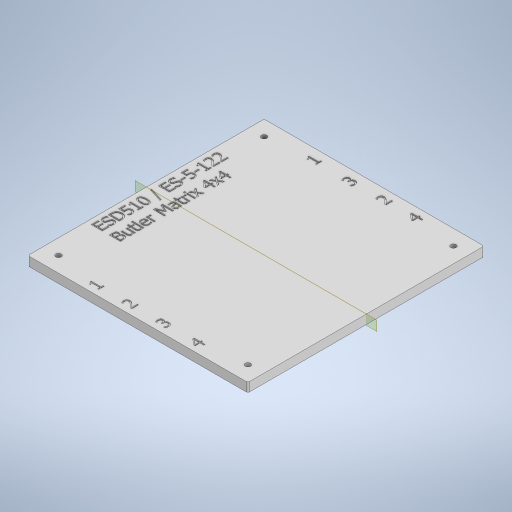
# Autodesk Inventor part: Cover_acryl
Saved by Autodesk Inventor 2023.5 (Build 275446000, 446)
## iProperties
Created: 2025-10-09
Part Number: Cover_acryl
Material: Generic
Document SubType Name: Modeling
Designer: Mikke
Density: 1 g/cm^3
Appearance: Default
Author: Mikke
Autodesk Inventor part; units mm, degrees
(part 1 of 2)
ref_plane "YZ Plane" through (0, 0, 0) normal (1, 0, 0) x (0, 1, 0)
ref_plane "XZ Plane" through (0, 0, 0) normal (0, 1, 0) x (-1, 0, 0)
ref_plane "XY Plane" through (0, 0, 0) normal (0, 0, 1) x (1, 0, 0)
sketch "Sketch1" plane through (0, 0, 0) normal (0, 1, 0) x (-1, 0, 0)
  line L0 (-61, 65.5) -> (61, 65.5)
  line L1 (61, 65.5) -> (61, -65.5)
  line L2 (61, -65.5) -> (-61, -65.5)
  line L3 (-61, -65.5) -> (-61, 65.5)
  line L4 (-61, 65.5) -> (61, -65.5) construction
  line L5 (61, 65.5) -> (-61, -65.5) construction
  point P0 (0, 0)
  dimension "d0" = 122
  dimension "d1" = 131
  constraints: 12 end point, 2 midpoint, 2 parallel, 1 horizontal, 1 perpendicular
  measures "d0" distance of L1.end L2.end
  measures "d1" distance of L0.end L1.end
extrude "Extrusion1" add sketch "Sketch1" along normal blind 5
sketch "Sketch2" plane through (0, 5, 0) normal (0, 1, 0) x (1, 0, 0)
  line L0 (-61, 65.5) -> (-61, -65.5) projected
  line L1 (-61, -65.5) -> (-52.5, -65.5)
  line L2 (-52.5, -65.5) -> (-52.5, -57)
  line L3 (-52.5, -57) -> (-61, -57)
  line L4 (-61, -57) -> (-61, -65.5)
  circle A0 centre (-52.5, -57) radius 1.5
  line L5 (-61, 65.5) -> (-61, -65.5) projected
  line L6 (-61, 65.5) -> (-52.5, 65.5)
  line L7 (-52.5, 65.5) -> (-52.5, 57)
  line L8 (-52.5, 57) -> (-61, 57)
  line L9 (-61, 57) -> (-61, 65.5)
  line L10 (61, 65.5) -> (-61, 65.5) projected
  line L11 (61, 65.5) -> (52.5, 65.5)
  line L12 (52.5, 65.5) -> (52.5, 57)
  line L13 (52.5, 57) -> (61, 57)
  line L14 (61, 57) -> (61, 65.5)
  line L15 (-61, -65.5) -> (61, -65.5) projected
  line L16 (61, -65.5) -> (52.5, -65.5)
  line L17 (52.5, -65.5) -> (52.5, -57)
  line L18 (52.5, -57) -> (61, -57)
  line L19 (61, -57) -> (61, -65.5)
  circle A1 centre (52.5, -57) radius 1.5
  circle A2 centre (52.5, 57) radius 1.5
  circle A3 centre (-52.5, 57) radius 1.5
  point P0 (0, 0)
  dimension "d4" = 8.5
  dimension "d5" = 8.5
  dimension "d6" = 3
  dimension "d7" = 8.5
  dimension "d8" = 8.5
  dimension "d9" = 8.5
  dimension "d10" = 8.5
  dimension "d11" = 8.5
  dimension "d12" = 8.5
  dimension "d13" = 3
  dimension "d14" = 3
  dimension "d15" = 3
  constraints: 32 end point, 8 parallel, 4 centre point, 4 coincident, 4 horizontal, 4 perpendicular
  measures "d4" distance of L3.end L2.end
  measures "d5" distance of L2.end L1.end
  measures "d6" diameter of A0
  measures "d7" distance of L7.end L8.end
  measures "d8" distance of L6.end L7.end
  measures "d9" distance of L13.end L12.end
  measures "d10" distance of L12.end L11.end
  measures "d11" distance of L17.end L18.end
  measures "d12" distance of L16.end L17.end
  measures "d13" diameter of A1
  measures "d14" diameter of A2
  measures "d15" diameter of A3
extrude "Extrusion2" cut sketch "Sketch2" against normal blind 5 contours A3 L7 L8 | L8 L7 A3 | A0 L2 L3 | L3 L2 A0 | A2 L13 L12 | L12 L13 A2 | A1 L18 L17 | L17 L18 A1
fillet "Fillet1" radius 1 4 edges at (61, 2.5, 65.5) (61, 2.5, -65.5) (-61, 2.5, -65.5) (-61, 2.5, 65.5)
sketch "Sketch4" plane through (0, 5, 0) normal (0, 1, 0) x (1, 0, 0)
  line L0 (-60, -65.5) -> (60, -65.5) projected
  line L1 (60, 65.5) -> (-60, 65.5) projected
  line L2 (0, -65.5) -> (-9.425, -65.5)
  line L3 (0, -65.5) -> (9.425, -65.5)
  line L4 (-9.425, -65.5) -> (-28.275, -65.5)
  line L5 (9.425, -65.5) -> (28.275, -65.5)
  line L6 (24.7297, -62.6951) -> (24.7297, -58.1177) construction
  line L7 (24.7297, -58.1177) -> (30.8297, -58.1177) construction
  line L8 (30.8297, -58.1177) -> (30.8297, -62.6951) construction
  line L9 (30.8297, -62.6951) -> (24.7297, -62.6951) construction
  line L10 (-31.1768, -63.0534) -> (-31.1768, -58.4759) construction
  line L11 (-31.1768, -58.4759) -> (-25.057, -58.4759) construction
  line L12 (-25.057, -58.4759) -> (-25.057, -63.0534) construction
  line L13 (-25.057, -63.0534) -> (-31.1768, -63.0534) construction
  line L14 (-12.8022, -62.7702) -> (-12.8022, -58.1927) construction
  line L15 (-12.8022, -58.1927) -> (-6.5737, -58.1927) construction
  line L16 (-6.5737, -58.1927) -> (-6.5737, -62.7702) construction
  line L17 (-6.5737, -62.7702) -> (-12.8022, -62.7702) construction
  line L18 (5.8471, -62.6329) -> (5.8471, -58.0555) construction
  line L19 (5.8471, -58.0555) -> (12.2041, -58.0555) construction
  line L20 (12.2041, -58.0555) -> (12.2041, -62.6329) construction
  line L21 (12.2041, -62.6329) -> (5.8471, -62.6329) construction
  line L22 (-28.275, -65.5) -> (-28.275, 65.5)
  line L23 (25.0797, 57.6837) -> (25.0797, 62.2611) construction
  line L24 (25.0797, 62.2611) -> (31.1797, 62.2611) construction
  line L25 (31.1797, 62.2611) -> (31.1797, 57.6837) construction
  line L26 (31.1797, 57.6837) -> (25.0797, 57.6837) construction
  line L27 (-30.8268, 57.3254) -> (-30.8268, 61.9029) construction
  line L28 (-30.8268, 61.9029) -> (-24.707, 61.9029) construction
  line L29 (-24.707, 61.9029) -> (-24.707, 57.3254) construction
  line L30 (-24.707, 57.3254) -> (-30.8268, 57.3254) construction
  line L31 (7.8308, 57.6086) -> (7.8308, 62.1861) construction
  line L32 (7.8308, 62.1861) -> (14.0593, 62.1861) construction
  line L33 (14.0593, 62.1861) -> (14.0593, 57.6086) construction
  line L34 (14.0593, 57.6086) -> (7.8308, 57.6086) construction
  line L35 (-10.5783, 57.1359) -> (-10.5783, 61.7133) construction
  line L36 (-10.5783, 61.7133) -> (-4.2212, 61.7133) construction
  line L37 (-4.2212, 61.7133) -> (-4.2212, 57.1359) construction
  line L38 (-4.2212, 57.1359) -> (-10.5783, 57.1359) construction
  line L39 (-25.057, -59.1531) -> (-25.057, -62.129)
  line L40 (-25.057, -62.129) -> (-25.6799, -62.129)
  line L41 (-25.6799, -62.129) -> (-25.6799, -61.0217)
  line L42 (-25.6799, -61.0217) -> (-29.768, -61.0217)
  line L43 (-29.768, -61.0217) -> (-29.768, -62.129)
  line L44 (-29.768, -62.129) -> (-30.3266, -62.129)
  spline S0 degree 2 poles (-30.3266, -62.129) (-30.3266, -61.5012) (-30.6825, -60.908) (-31.1768, -60.8684) knots 0 0 0 1 2 2 2
  line L45 (-31.1768, -60.8684) -> (-31.1768, -60.2357)
  line L46 (-31.1768, -60.2357) -> (-25.6799, -60.2357)
  line L47 (-25.6799, -60.2357) -> (-25.6799, -59.1531)
  line L48 (-25.6799, -59.1531) -> (-25.057, -59.1531)
  line L49 (-6.5737, -58.5635) -> (-6.5737, -62.3253)
  line L50 (-6.5737, -62.3253) -> (-7.4388, -62.3253)
  spline S1 degree 2 poles (-7.4388, -62.3253) (-7.8194, -61.9199) (-8.5263, -61.1982) (-8.9069, -60.8522) knots 0 0 0 1 2 2 2
  spline S2 degree 2 poles (-8.9069, -60.8522) (-9.6731, -60.1552) (-10.5926, -59.646) (-11.0819, -59.646) knots 0 0 0 1 2 2 2
  spline S3 degree 2 poles (-11.0819, -59.646) (-11.339, -59.646) (-11.7246, -59.8042) (-11.8482, -59.9476) knots 0 0 0 1 2 2 2
  spline S4 degree 2 poles (-11.8482, -59.9476) (-11.9717, -60.0909) (-12.0953, -60.4666) (-12.0953, -60.694) knots 0 0 0 1 2 2 2
  spline S5 degree 2 poles (-12.0953, -60.694) (-12.0953, -60.9115) (-11.9866, -61.3564) (-11.9025, -61.5591) knots 0 0 0 1 2 2 2
  spline S6 degree 2 poles (-11.9025, -61.5591) (-11.8333, -61.7321) (-11.6356, -62.0534) (-11.5664, -62.1523) knots 0 0 0 1 2 2 2
  line L51 (-11.5664, -62.1523) -> (-11.5664, -62.1968)
  line L52 (-11.5664, -62.1968) -> (-12.4364, -62.1968)
  spline S7 degree 2 poles (-12.4364, -62.1968) (-12.56, -61.9447) (-12.8022, -61.04) (-12.8022, -60.6347) knots 0 0 0 1 2 2 2
  spline S8 degree 2 poles (-12.8022, -60.6347) (-12.8022, -59.7795) (-11.8976, -58.8156) (-11.1264, -58.8156) knots 0 0 0 1 2 2 2
  spline S9 degree 2 poles (-11.1264, -58.8156) (-10.7656, -58.8156) (-10.1625, -58.9836) (-9.9054, -59.1319) knots 0 0 0 1 2 2 2
  spline S10 degree 2 poles (-9.9054, -59.1319) (-9.6385, -59.2802) (-9.1145, -59.7103) (-8.8624, -59.9476) knots 0 0 0 1 2 2 2
  spline S11 degree 2 poles (-8.8624, -59.9476) (-8.4422, -60.3331) (-7.5426, -61.2773) (-7.2806, -61.5591) knots 0 0 0 1 2 2 2
  line L53 (-7.2806, -61.5591) -> (-7.2806, -58.5635)
  line L54 (-7.2806, -58.5635) -> (-6.5737, -58.5635)
  spline S12 degree 2 poles (6.554, -60.5419) (6.554, -60.7644) (6.6627, -61.2043) (6.7467, -61.4169) knots 0 0 0 1 2 2 2
  spline S13 degree 2 poles (6.7467, -61.4169) (6.8308, -61.6146) (7.0087, -61.9063) (7.0878, -62.02) knots 0 0 0 1 2 2 2
  line L55 (7.0878, -62.02) -> (7.0878, -62.0694)
  line L56 (7.0878, -62.0694) -> (6.2228, -62.0694)
  spline S14 degree 2 poles (6.2228, -62.0694) (6.0794, -61.8025) (5.8471, -60.888) (5.8471, -60.4777) knots 0 0 0 1 2 2 2
  spline S15 degree 2 poles (5.8471, -60.4777) (5.8471, -60.0624) (6.0151, -59.4445) (6.1931, -59.1924) knots 0 0 0 1 2 2 2
  spline S16 degree 2 poles (6.1931, -59.1924) (6.3859, -58.9255) (6.9445, -58.6487) (7.3202, -58.6487) knots 0 0 0 1 2 2 2
  spline S17 degree 2 poles (7.3202, -58.6487) (7.8244, -58.6487) (8.5856, -59.3111) (8.6845, -59.7757) knots 0 0 0 1 2 2 2
  line L57 (8.6845, -59.7757) -> (8.7438, -59.7757)
  spline S18 degree 2 poles (8.7438, -59.7757) (8.7834, -59.5829) (8.9613, -59.143) (9.1393, -58.9551) knots 0 0 0 1 2 2 2
  spline S19 degree 2 poles (9.1393, -58.9551) (9.3123, -58.7673) (9.866, -58.53) (10.2664, -58.53) knots 0 0 0 1 2 2 2
  spline S20 degree 2 poles (10.2664, -58.53) (10.6767, -58.53) (11.3737, -58.8118) (11.6406, -59.0688) knots 0 0 0 1 2 2 2
  spline S21 degree 2 poles (11.6406, -59.0688) (11.9174, -59.3358) (12.2041, -60.0921) (12.2041, -60.5716) knots 0 0 0 1 2 2 2
  spline S22 degree 2 poles (12.2041, -60.5716) (12.2041, -61.0313) (11.9817, -61.931) (11.8284, -62.2375) knots 0 0 0 1 2 2 2
  line L58 (11.8284, -62.2375) -> (10.9634, -62.2375)
  line L59 (10.9634, -62.2375) -> (10.9634, -62.1782)
  spline S23 degree 2 poles (10.9634, -62.1782) (11.1512, -61.9211) (11.4972, -61.0511) (11.4972, -60.621) knots 0 0 0 1 2 2 2
  spline S24 degree 2 poles (11.4972, -60.621) (11.4972, -60.3689) (11.339, -59.8647) (11.1561, -59.6966) knots 0 0 0 1 2 2 2
  spline S25 degree 2 poles (11.1561, -59.6966) (10.9732, -59.5335) (10.5382, -59.3605) (10.207, -59.3605) knots 0 0 0 1 2 2 2
  spline S26 degree 2 poles (10.207, -59.3605) (9.8758, -59.3605) (9.4458, -59.5533) (9.3222, -59.7263) knots 0 0 0 1 2 2 2
  spline S27 degree 2 poles (9.3222, -59.7263) (9.1986, -59.8993) (9.1047, -60.3689) (9.1047, -60.6457) knots 0 0 0 1 2 2 2
  line L60 (9.1047, -60.6457) -> (9.1047, -60.9918)
  line L61 (9.1047, -60.9918) -> (8.4275, -60.9918)
  line L62 (8.4275, -60.9918) -> (8.4275, -60.7199)
  spline S28 degree 2 poles (8.4275, -60.7199) (8.4275, -60.1712) (7.9035, -59.4791) (7.4042, -59.4791) knots 0 0 0 1 2 2 2
  spline S29 degree 2 poles (7.4042, -59.4791) (7.1719, -59.4791) (6.8407, -59.6571) (6.7418, -59.8004) knots 0 0 0 1 2 2 2
  spline S30 degree 2 poles (6.7418, -59.8004) (6.638, -59.9537) (6.554, -60.3294) (6.554, -60.5419) knots 0 0 0 1 2 2 2
  line L63 (28.7338, -58.3253) -> (28.7338, -59.0519)
  line L64 (28.7338, -59.0519) -> (30.8297, -59.0519)
  line L65 (30.8297, -59.0519) -> (30.8297, -59.8379)
  line L66 (30.8297, -59.8379) -> (28.7338, -59.8379)
  line L67 (28.7338, -59.8379) -> (28.7338, -62.532)
  line L68 (28.7338, -62.532) -> (27.8736, -62.532)
  line L69 (27.8736, -62.532) -> (24.7297, -59.8033)
  line L70 (24.7297, -59.8033) -> (24.7297, -59.0519)
  line L71 (24.7297, -59.0519) -> (28.0763, -59.0519)
  line L72 (28.0763, -59.0519) -> (28.0763, -58.3253)
  line L73 (28.0763, -58.3253) -> (28.7338, -58.3253)
  line L74 (28.0763, -59.8379) -> (25.6937, -59.8379)
  line L75 (25.6937, -59.8379) -> (28.0763, -61.8894)
  line L76 (28.0763, -61.8894) -> (28.0763, -59.8379)
  line L77 (-24.707, 61.2257) -> (-24.707, 58.2498)
  line L78 (-24.707, 58.2498) -> (-25.3299, 58.2498)
  line L79 (-25.3299, 58.2498) -> (-25.3299, 59.3571)
  line L80 (-25.3299, 59.3571) -> (-29.418, 59.3571)
  line L81 (-29.418, 59.3571) -> (-29.418, 58.2498)
  line L82 (-29.418, 58.2498) -> (-29.9765, 58.2498)
  spline S31 degree 2 poles (-29.9765, 58.2498) (-29.9765, 58.8776) (-30.3325, 59.4708) (-30.8268, 59.5104) knots 0 0 0 1 2 2 2
  line L83 (-30.8268, 59.5104) -> (-30.8268, 60.1431)
  line L84 (-30.8268, 60.1431) -> (-25.3299, 60.1431)
  line L85 (-25.3299, 60.1431) -> (-25.3299, 61.2257)
  line L86 (-25.3299, 61.2257) -> (-24.707, 61.2257)
  line L87 (14.0593, 61.8154) -> (14.0593, 58.0535)
  line L88 (14.0593, 58.0535) -> (13.1942, 58.0535)
  spline S32 degree 2 poles (13.1942, 58.0535) (12.8136, 58.4589) (12.1067, 59.1806) (11.7261, 59.5266) knots 0 0 0 1 2 2 2
  spline S33 degree 2 poles (11.7261, 59.5266) (10.9599, 60.2236) (10.0404, 60.7328) (9.551, 60.7328) knots 0 0 0 1 2 2 2
  spline S34 degree 2 poles (9.551, 60.7328) (9.294, 60.7328) (8.9084, 60.5746) (8.7848, 60.4312) knots 0 0 0 1 2 2 2
  spline S35 degree 2 poles (8.7848, 60.4312) (8.6612, 60.2879) (8.5377, 59.9122) (8.5377, 59.6848) knots 0 0 0 1 2 2 2
  spline S36 degree 2 poles (8.5377, 59.6848) (8.5377, 59.4673) (8.6464, 59.0224) (8.7305, 58.8197) knots 0 0 0 1 2 2 2
  spline S37 degree 2 poles (8.7305, 58.8197) (8.7997, 58.6467) (8.9974, 58.3254) (9.0666, 58.2265) knots 0 0 0 1 2 2 2
  line L89 (9.0666, 58.2265) -> (9.0666, 58.1821)
  line L90 (9.0666, 58.1821) -> (8.1966, 58.1821)
  spline S38 degree 2 poles (8.1966, 58.1821) (8.073, 58.4342) (7.8308, 59.3388) (7.8308, 59.7441) knots 0 0 0 1 2 2 2
  spline S39 degree 2 poles (7.8308, 59.7441) (7.8308, 60.5993) (8.7354, 61.5633) (9.5065, 61.5633) knots 0 0 0 1 2 2 2
  spline S40 degree 2 poles (9.5065, 61.5633) (9.8674, 61.5633) (10.4705, 61.3952) (10.7275, 61.2469) knots 0 0 0 1 2 2 2
  spline S41 degree 2 poles (10.7275, 61.2469) (10.9945, 61.0986) (11.5185, 60.6685) (11.7706, 60.4312) knots 0 0 0 1 2 2 2
  spline S42 degree 2 poles (11.7706, 60.4312) (12.1907, 60.0457) (13.0904, 59.1015) (13.3524, 58.8197) knots 0 0 0 1 2 2 2
  line L91 (13.3524, 58.8197) -> (13.3524, 61.8154)
  line L92 (13.3524, 61.8154) -> (14.0593, 61.8154)
  spline S43 degree 2 poles (-9.8714, 59.2269) (-9.8714, 59.0044) (-9.7627, 58.5645) (-9.6786, 58.3519) knots 0 0 0 1 2 2 2
  spline S44 degree 2 poles (-9.6786, 58.3519) (-9.5946, 58.1542) (-9.4166, 57.8625) (-9.3375, 57.7488) knots 0 0 0 1 2 2 2
  line L93 (-9.3375, 57.7488) -> (-9.3375, 57.6994)
  line L94 (-9.3375, 57.6994) -> (-10.2026, 57.6994)
  spline S45 degree 2 poles (-10.2026, 57.6994) (-10.346, 57.9663) (-10.5783, 58.8808) (-10.5783, 59.2911) knots 0 0 0 1 2 2 2
  spline S46 degree 2 poles (-10.5783, 59.2911) (-10.5783, 59.7064) (-10.4102, 60.3243) (-10.2323, 60.5764) knots 0 0 0 1 2 2 2
  spline S47 degree 2 poles (-10.2323, 60.5764) (-10.0395, 60.8433) (-9.4809, 61.1201) (-9.1052, 61.1201) knots 0 0 0 1 2 2 2
  spline S48 degree 2 poles (-9.1052, 61.1201) (-8.601, 61.1201) (-7.8397, 60.4577) (-7.7409, 59.9931) knots 0 0 0 1 2 2 2
  line L95 (-7.7409, 59.9931) -> (-7.6815, 59.9931)
  spline S49 degree 2 poles (-7.6815, 59.9931) (-7.642, 60.1859) (-7.464, 60.6258) (-7.2861, 60.8137) knots 0 0 0 1 2 2 2
  spline S50 degree 2 poles (-7.2861, 60.8137) (-7.1131, 61.0015) (-6.5594, 61.2388) (-6.159, 61.2388) knots 0 0 0 1 2 2 2
  spline S51 degree 2 poles (-6.159, 61.2388) (-5.7487, 61.2388) (-5.0517, 60.957) (-4.7848, 60.7) knots 0 0 0 1 2 2 2
  spline S52 degree 2 poles (-4.7848, 60.7) (-4.508, 60.433) (-4.2212, 59.6767) (-4.2212, 59.1972) knots 0 0 0 1 2 2 2
  spline S53 degree 2 poles (-4.2212, 59.1972) (-4.2212, 58.7375) (-4.4437, 57.8378) (-4.5969, 57.5313) knots 0 0 0 1 2 2 2
  line L96 (-4.5969, 57.5313) -> (-5.462, 57.5313)
  line L97 (-5.462, 57.5313) -> (-5.462, 57.5906)
  spline S54 degree 2 poles (-5.462, 57.5906) (-5.2742, 57.8477) (-4.9281, 58.7177) (-4.9281, 59.1478) knots 0 0 0 1 2 2 2
  spline S55 degree 2 poles (-4.9281, 59.1478) (-4.9281, 59.3999) (-5.0863, 59.9041) (-5.2692, 60.0722) knots 0 0 0 1 2 2 2
  spline S56 degree 2 poles (-5.2692, 60.0722) (-5.4521, 60.2353) (-5.8871, 60.4083) (-6.2183, 60.4083) knots 0 0 0 1 2 2 2
  spline S57 degree 2 poles (-6.2183, 60.4083) (-6.5495, 60.4083) (-6.9796, 60.2155) (-7.1032, 60.0425) knots 0 0 0 1 2 2 2
  spline S58 degree 2 poles (-7.1032, 60.0425) (-7.2268, 59.8695) (-7.3207, 59.3999) (-7.3207, 59.1231) knots 0 0 0 1 2 2 2
  line L98 (-7.3207, 59.1231) -> (-7.3207, 58.777)
  line L99 (-7.3207, 58.777) -> (-7.9979, 58.777)
  line L100 (-7.9979, 58.777) -> (-7.9979, 59.0489)
  spline S59 degree 2 poles (-7.9979, 59.0489) (-7.9979, 59.5976) (-8.5219, 60.2897) (-9.0212, 60.2897) knots 0 0 0 1 2 2 2
  spline S60 degree 2 poles (-9.0212, 60.2897) (-9.2535, 60.2897) (-9.5847, 60.1117) (-9.6836, 59.9684) knots 0 0 0 1 2 2 2
  spline S61 degree 2 poles (-9.6836, 59.9684) (-9.7874, 59.8151) (-9.8714, 59.4394) (-9.8714, 59.2269) knots 0 0 0 1 2 2 2
  line L101 (29.0838, 62.0535) -> (29.0838, 61.3269)
  line L102 (29.0838, 61.3269) -> (31.1797, 61.3269)
  line L103 (31.1797, 61.3269) -> (31.1797, 60.5409)
  line L104 (31.1797, 60.5409) -> (29.0838, 60.5409)
  line L105 (29.0838, 60.5409) -> (29.0838, 57.8468)
  line L106 (29.0838, 57.8468) -> (28.2237, 57.8468)
  line L107 (28.2237, 57.8468) -> (25.0797, 60.5755)
  line L108 (25.0797, 60.5755) -> (25.0797, 61.3269)
  line L109 (25.0797, 61.3269) -> (28.4263, 61.3269)
  line L110 (28.4263, 61.3269) -> (28.4263, 62.0535)
  line L111 (28.4263, 62.0535) -> (29.0838, 62.0535)
  line L112 (28.4263, 60.5409) -> (26.0437, 60.5409)
  line L113 (26.0437, 60.5409) -> (28.4263, 58.4894)
  line L114 (28.4263, 58.4894) -> (28.4263, 60.5409)
  point P0 (0, 0)
  point P1 (0, 65.5)
  dimension "d19" = 9.425
  dimension "d20" = 9.425
  dimension "d21" = 18.85
  dimension "d22" = 18.85
  constraints: 10 end point, 5 point on line, 2 midpoint, 1 perpendicular, 16 other
  measures "d19" distance of L2.start L2.end
  measures "d20" distance of L2.start L3.end
  measures "d21" distance of L2.end L4.end
  measures "d22" distance of L3.end L5.end
extrude "Extrusion4" cut sketch "Sketch4" against normal blind 0.5
ref_plane "Work Plane1" through (60, 0, 0) normal (0, 0, -1) x (-1, 0, 0)
sketch "Sketch5" plane through (0, 5, 0) normal (0, 1, 0) x (1, 0, 0)
  line L0 (-58.5499, -33.7379) -> (-58.5499, 37.287) construction
  line L1 (-58.5499, 37.287) -> (-42.006, 37.287) construction
  line L2 (-42.006, 37.287) -> (-42.006, -33.7379) construction
  line L3 (-42.006, -33.7379) -> (-58.5499, -33.7379) construction
  line L4 (-52.178, -33.12) -> (-58.278, -33.12)
  line L5 (-58.278, -33.12) -> (-58.278, -29.3038)
  line L6 (-58.278, -29.3038) -> (-57.5563, -29.3038)
  line L7 (-57.5563, -29.3038) -> (-57.5563, -32.3093)
  line L8 (-57.5563, -32.3093) -> (-55.8855, -32.3093)
  line L9 (-55.8855, -32.3093) -> (-55.8855, -29.5065)
  line L10 (-55.8855, -29.5065) -> (-55.1637, -29.5065)
  line L11 (-55.1637, -29.5065) -> (-55.1637, -32.3093)
  line L12 (-55.1637, -32.3093) -> (-52.8997, -32.3093)
  line L13 (-52.8997, -32.3093) -> (-52.8997, -29.3038)
  line L14 (-52.8997, -29.3038) -> (-52.178, -29.3038)
  line L15 (-52.178, -29.3038) -> (-52.178, -33.12)
  spline S0 degree 2 poles (-52.0692, -26.7135) (-52.0692, -27.3759) (-52.3461, -28.3053) (-52.5438, -28.7156) knots 0 0 0 1 2 2 2
  line L16 (-52.5438, -28.7156) -> (-53.5621, -28.7156)
  line L17 (-53.5621, -28.7156) -> (-53.5621, -28.6562)
  spline S1 degree 2 poles (-53.5621, -28.6562) (-53.1864, -28.2558) (-52.7712, -27.2425) (-52.7712, -26.7729) knots 0 0 0 1 2 2 2
  spline S2 degree 2 poles (-52.7712, -26.7729) (-52.7712, -26.1006) (-53.3298, -25.4135) (-53.7895, -25.4135) knots 0 0 0 1 2 2 2
  spline S3 degree 2 poles (-53.7895, -25.4135) (-54.1553, -25.4135) (-54.6101, -25.7743) (-54.7238, -26.1648) knots 0 0 0 1 2 2 2
  spline S4 degree 2 poles (-54.7238, -26.1648) (-54.8029, -26.4466) (-54.9116, -26.9162) (-55.0006, -27.2672) knots 0 0 0 1 2 2 2
  spline S5 degree 2 poles (-55.0006, -27.2672) (-55.0846, -27.5836) (-55.3367, -28.0828) (-55.5394, -28.2756) knots 0 0 0 1 2 2 2
  spline S6 degree 2 poles (-55.5394, -28.2756) (-55.7421, -28.4635) (-56.2859, -28.6711) (-56.6418, -28.6711) knots 0 0 0 1 2 2 2
  spline S7 degree 2 poles (-56.6418, -28.6711) (-57.3833, -28.6711) (-58.3867, -27.5144) (-58.3867, -26.6196) knots 0 0 0 1 2 2 2
  spline S8 degree 2 poles (-58.3867, -26.6196) (-58.3867, -26.1055) (-58.1841, -25.196) (-57.9913, -24.8054) knots 0 0 0 1 2 2 2
  line L18 (-57.9913, -24.8054) -> (-57.0224, -24.8054)
  line L19 (-57.0224, -24.8054) -> (-57.0224, -24.8648)
  spline S9 degree 2 poles (-57.0224, -24.8648) (-57.2893, -25.1564) (-57.6848, -26.066) (-57.6848, -26.5652) knots 0 0 0 1 2 2 2
  spline S10 degree 2 poles (-57.6848, -26.5652) (-57.6848, -27.1288) (-57.1559, -27.8258) (-56.7258, -27.8258) knots 0 0 0 1 2 2 2
  spline S11 degree 2 poles (-56.7258, -27.8258) (-56.3402, -27.8258) (-55.8805, -27.4155) (-55.7767, -27.0299) knots 0 0 0 1 2 2 2
  spline S12 degree 2 poles (-55.7767, -27.0299) (-55.7075, -26.7729) (-55.5295, -26.0264) (-55.4554, -25.7793) knots 0 0 0 1 2 2 2
  spline S13 degree 2 poles (-55.4554, -25.7793) (-55.2626, -25.1515) (-54.4865, -24.5682) (-53.918, -24.5682) knots 0 0 0 1 2 2 2
  spline S14 degree 2 poles (-53.918, -24.5682) (-53.5572, -24.5682) (-52.8651, -24.8598) (-52.6229, -25.1218) knots 0 0 0 1 2 2 2
  spline S15 degree 2 poles (-52.6229, -25.1218) (-52.356, -25.4135) (-52.0692, -26.155) (-52.0692, -26.7135) knots 0 0 0 1 2 2 2
  spline S16 degree 2 poles (-55.2231, -18.9328) (-54.3876, -18.9328) (-53.0431, -19.6101) (-52.6674, -20.1785) knots 0 0 0 1 2 2 2
  spline S17 degree 2 poles (-52.6674, -20.1785) (-52.3757, -20.6432) (-52.178, -21.5973) (-52.178, -22.3387) knots 0 0 0 1 2 2 2
  line L20 (-52.178, -22.3387) -> (-52.178, -23.7426)
  line L21 (-52.178, -23.7426) -> (-58.278, -23.7426)
  line L22 (-58.278, -23.7426) -> (-58.278, -22.3536)
  spline S18 degree 2 poles (-58.278, -22.3536) (-58.278, -21.4934) (-58.0209, -20.5147) (-57.7936, -20.1686) knots 0 0 0 1 2 2 2
  spline S19 degree 2 poles (-57.7936, -20.1686) (-57.403, -19.5804) (-56.1128, -18.9328) (-55.2231, -18.9328) knots 0 0 0 1 2 2 2
  spline S20 degree 2 poles (-55.2329, -19.7781) (-55.9349, -19.7781) (-56.9285, -20.2428) (-57.2102, -20.7025) knots 0 0 0 1 2 2 2
  spline S21 degree 2 poles (-57.2102, -20.7025) (-57.403, -21.0288) (-57.5761, -21.7653) (-57.5761, -22.314) knots 0 0 0 1 2 2 2
  line L23 (-57.5761, -22.314) -> (-57.5761, -22.9319)
  line L24 (-57.5761, -22.9319) -> (-52.8799, -22.9319)
  line L25 (-52.8799, -22.9319) -> (-52.8799, -22.314)
  spline S22 degree 2 poles (-52.8799, -22.314) (-52.8799, -21.7752) (-53.053, -20.9596) (-53.2853, -20.6284) knots 0 0 0 1 2 2 2
  spline S23 degree 2 poles (-53.2853, -20.6284) (-53.572, -20.2032) (-54.5211, -19.7781) (-55.2329, -19.7781) knots 0 0 0 1 2 2 2
  spline S24 degree 2 poles (-54.1158, -14.5284) (-53.6758, -14.5284) (-52.9244, -14.8101) (-52.6476, -15.0672) knots 0 0 0 1 2 2 2
  spline S25 degree 2 poles (-52.6476, -15.0672) (-52.3708, -15.3242) (-52.0495, -16.0904) (-52.0495, -16.565) knots 0 0 0 1 2 2 2
  spline S26 degree 2 poles (-52.0495, -16.565) (-52.0495, -17) (-52.2423, -17.8503) (-52.3955, -18.1617) knots 0 0 0 1 2 2 2
  line L26 (-52.3955, -18.1617) -> (-53.2606, -18.1617)
  line L27 (-53.2606, -18.1617) -> (-53.2606, -18.1024)
  spline S27 degree 2 poles (-53.2606, -18.1024) (-53.1914, -18.0084) (-53.0134, -17.6575) (-52.9343, -17.4449) knots 0 0 0 1 2 2 2
  spline S28 degree 2 poles (-52.9343, -17.4449) (-52.8503, -17.2027) (-52.7564, -16.8023) (-52.7564, -16.5502) knots 0 0 0 1 2 2 2
  spline S29 degree 2 poles (-52.7564, -16.5502) (-52.7564, -16.303) (-52.9343, -15.8383) (-53.1271, -15.6703) knots 0 0 0 1 2 2 2
  spline S30 degree 2 poles (-53.1271, -15.6703) (-53.31, -15.517) (-53.7944, -15.3588) (-54.1207, -15.3588) knots 0 0 0 1 2 2 2
  spline S31 degree 2 poles (-54.1207, -15.3588) (-54.447, -15.3588) (-54.8622, -15.5368) (-55.0006, -15.7049) knots 0 0 0 1 2 2 2
  spline S32 degree 2 poles (-55.0006, -15.7049) (-55.1538, -15.8779) (-55.2824, -16.392) (-55.2824, -16.7034) knots 0 0 0 1 2 2 2
  spline S33 degree 2 poles (-55.2824, -16.7034) (-55.2824, -17.0396) (-55.1786, -17.7069) (-55.1341, -17.9096) knots 0 0 0 1 2 2 2
  line L28 (-55.1341, -17.9096) -> (-58.278, -17.9096)
  line L29 (-58.278, -17.9096) -> (-58.278, -14.563)
  line L30 (-58.278, -14.563) -> (-57.5612, -14.563)
  line L31 (-57.5612, -14.563) -> (-57.5612, -17.1236)
  line L32 (-57.5612, -17.1236) -> (-55.9349, -17.1236)
  spline S34 degree 2 poles (-55.9349, -17.1236) (-55.9547, -16.9753) (-55.9695, -16.6886) (-55.9695, -16.5699) knots 0 0 0 1 2 2 2
  spline S35 degree 2 poles (-55.9695, -16.5699) (-55.9695, -16.1003) (-55.8162, -15.4528) (-55.5889, -15.1562) knots 0 0 0 1 2 2 2
  spline S36 degree 2 poles (-55.5889, -15.1562) (-55.3615, -14.8546) (-54.6694, -14.5284) (-54.1158, -14.5284) knots 0 0 0 1 2 2 2
  line L33 (-52.178, -10.1931) -> (-52.178, -13.169)
  line L34 (-52.178, -13.169) -> (-52.8008, -13.169)
  line L35 (-52.8008, -13.169) -> (-52.8008, -12.0617)
  line L36 (-52.8008, -12.0617) -> (-56.8889, -12.0617)
  line L37 (-56.8889, -12.0617) -> (-56.8889, -13.169)
  line L38 (-56.8889, -13.169) -> (-57.4475, -13.169)
  spline S37 degree 2 poles (-57.4475, -13.169) (-57.4475, -12.5412) (-57.8034, -11.948) (-58.2978, -11.9084) knots 0 0 0 1 2 2 2
  line L39 (-58.2978, -11.9084) -> (-58.2978, -11.2757)
  line L40 (-58.2978, -11.2757) -> (-52.8008, -11.2757)
  line L41 (-52.8008, -11.2757) -> (-52.8008, -10.1931)
  line L42 (-52.8008, -10.1931) -> (-52.178, -10.1931)
  spline S38 degree 2 poles (-55.228, -5.2746) (-53.5868, -5.2746) (-52.0495, -6.2286) (-52.0495, -7.2222) knots 0 0 0 1 2 2 2
  spline S39 degree 2 poles (-52.0495, -7.2222) (-52.0495, -8.2306) (-53.6165, -9.1748) (-55.2231, -9.1748) knots 0 0 0 1 2 2 2
  spline S40 degree 2 poles (-55.2231, -9.1748) (-56.8741, -9.1748) (-58.4016, -8.2208) (-58.4016, -7.2222) knots 0 0 0 1 2 2 2
  spline S41 degree 2 poles (-58.4016, -7.2222) (-58.4016, -6.2187) (-56.8197, -5.2746) (-55.228, -5.2746) knots 0 0 0 1 2 2 2
  spline S42 degree 2 poles (-53.3693, -6.3225) (-53.6709, -6.2039) (-54.6002, -6.105) (-55.228, -6.105) knots 0 0 0 1 2 2 2
  spline S43 degree 2 poles (-55.228, -6.105) (-55.8558, -6.105) (-56.7802, -6.2039) (-57.0916, -6.3275) knots 0 0 0 1 2 2 2
  spline S44 degree 2 poles (-57.0916, -6.3275) (-57.403, -6.4511) (-57.7243, -6.8811) (-57.7243, -7.2222) knots 0 0 0 1 2 2 2
  spline S45 degree 2 poles (-57.7243, -7.2222) (-57.7243, -7.5633) (-57.403, -8.0032) (-57.0817, -8.1318) knots 0 0 0 1 2 2 2
  spline S46 degree 2 poles (-57.0817, -8.1318) (-56.7703, -8.2554) (-55.8212, -8.3443) (-55.2231, -8.3443) knots 0 0 0 1 2 2 2
  spline S47 degree 2 poles (-55.2231, -8.3443) (-54.5804, -8.3443) (-53.7203, -8.2652) (-53.3842, -8.1367) knots 0 0 0 1 2 2 2
  spline S48 degree 2 poles (-53.3842, -8.1367) (-53.0678, -8.0181) (-52.7267, -7.5781) (-52.7267, -7.2222) knots 0 0 0 1 2 2 2
  spline S49 degree 2 poles (-52.7267, -7.2222) (-52.7267, -6.8861) (-53.048, -6.4461) (-53.3693, -6.3225) knots 0 0 0 1 2 2 2
  line L43 (-58.5499, 0.6623) -> (-50.8532, -1.7253)
  line L44 (-50.8532, -1.7253) -> (-50.8532, -2.4173)
  line L45 (-50.8532, -2.4173) -> (-58.5499, -0.0396)
  line L46 (-58.5499, -0.0396) -> (-58.5499, 0.6623)
  line L47 (-52.178, 4.1275) -> (-58.278, 4.1275)
  line L48 (-58.278, 4.1275) -> (-58.278, 7.9438)
  line L49 (-58.278, 7.9438) -> (-57.5563, 7.9438)
  line L50 (-57.5563, 7.9438) -> (-57.5563, 4.9382)
  line L51 (-57.5563, 4.9382) -> (-55.8855, 4.9382)
  line L52 (-55.8855, 4.9382) -> (-55.8855, 7.7411)
  line L53 (-55.8855, 7.7411) -> (-55.1637, 7.7411)
  line L54 (-55.1637, 7.7411) -> (-55.1637, 4.9382)
  line L55 (-55.1637, 4.9382) -> (-52.8997, 4.9382)
  line L56 (-52.8997, 4.9382) -> (-52.8997, 7.9438)
  line L57 (-52.8997, 7.9438) -> (-52.178, 7.9438)
  line L58 (-52.178, 7.9438) -> (-52.178, 4.1275)
  spline S50 degree 2 poles (-52.0692, 10.534) (-52.0692, 9.8716) (-52.3461, 8.9423) (-52.5438, 8.532) knots 0 0 0 1 2 2 2
  line L59 (-52.5438, 8.532) -> (-53.5621, 8.532)
  line L60 (-53.5621, 8.532) -> (-53.5621, 8.5913)
  spline S51 degree 2 poles (-53.5621, 8.5913) (-53.1864, 8.9917) (-52.7712, 10.0051) (-52.7712, 10.4747) knots 0 0 0 1 2 2 2
  spline S52 degree 2 poles (-52.7712, 10.4747) (-52.7712, 11.147) (-53.3298, 11.8341) (-53.7895, 11.8341) knots 0 0 0 1 2 2 2
  spline S53 degree 2 poles (-53.7895, 11.8341) (-54.1553, 11.8341) (-54.6101, 11.4733) (-54.7238, 11.0827) knots 0 0 0 1 2 2 2
  spline S54 degree 2 poles (-54.7238, 11.0827) (-54.8029, 10.801) (-54.9116, 10.3314) (-55.0006, 9.9804) knots 0 0 0 1 2 2 2
  spline S55 degree 2 poles (-55.0006, 9.9804) (-55.0846, 9.664) (-55.3367, 9.1647) (-55.5394, 8.972) knots 0 0 0 1 2 2 2
  spline S56 degree 2 poles (-55.5394, 8.972) (-55.7421, 8.7841) (-56.2859, 8.5765) (-56.6418, 8.5765) knots 0 0 0 1 2 2 2
  spline S57 degree 2 poles (-56.6418, 8.5765) (-57.3833, 8.5765) (-58.3867, 9.7332) (-58.3867, 10.628) knots 0 0 0 1 2 2 2
  spline S58 degree 2 poles (-58.3867, 10.628) (-58.3867, 11.1421) (-58.1841, 12.0516) (-57.9913, 12.4421) knots 0 0 0 1 2 2 2
  line L61 (-57.9913, 12.4421) -> (-57.0224, 12.4421)
  line L62 (-57.0224, 12.4421) -> (-57.0224, 12.3828)
  spline S59 degree 2 poles (-57.0224, 12.3828) (-57.2893, 12.0912) (-57.6848, 11.1816) (-57.6848, 10.6823) knots 0 0 0 1 2 2 2
  spline S60 degree 2 poles (-57.6848, 10.6823) (-57.6848, 10.1188) (-57.1559, 9.4218) (-56.7258, 9.4218) knots 0 0 0 1 2 2 2
  spline S61 degree 2 poles (-56.7258, 9.4218) (-56.3402, 9.4218) (-55.8805, 9.8321) (-55.7767, 10.2177) knots 0 0 0 1 2 2 2
  spline S62 degree 2 poles (-55.7767, 10.2177) (-55.7075, 10.4747) (-55.5295, 11.2211) (-55.4554, 11.4683) knots 0 0 0 1 2 2 2
  spline S63 degree 2 poles (-55.4554, 11.4683) (-55.2626, 12.0961) (-54.4865, 12.6794) (-53.918, 12.6794) knots 0 0 0 1 2 2 2
  spline S64 degree 2 poles (-53.918, 12.6794) (-53.5572, 12.6794) (-52.8651, 12.3878) (-52.6229, 12.1258) knots 0 0 0 1 2 2 2
  spline S65 degree 2 poles (-52.6229, 12.1258) (-52.356, 11.8341) (-52.0692, 11.0926) (-52.0692, 10.534) knots 0 0 0 1 2 2 2
  line L63 (-54.4766, 15.5663) -> (-54.4766, 13.2578)
  line L64 (-54.4766, 13.2578) -> (-55.2181, 13.2578)
  line L65 (-55.2181, 13.2578) -> (-55.2181, 15.5663)
  line L66 (-55.2181, 15.5663) -> (-54.4766, 15.5663)
  spline S66 degree 2 poles (-54.1158, 20.0745) (-53.6758, 20.0745) (-52.9244, 19.7928) (-52.6476, 19.5357) knots 0 0 0 1 2 2 2
  spline S67 degree 2 poles (-52.6476, 19.5357) (-52.3708, 19.2787) (-52.0495, 18.5125) (-52.0495, 18.0379) knots 0 0 0 1 2 2 2
  spline S68 degree 2 poles (-52.0495, 18.0379) (-52.0495, 17.6029) (-52.2423, 16.7527) (-52.3955, 16.4412) knots 0 0 0 1 2 2 2
  line L67 (-52.3955, 16.4412) -> (-53.2606, 16.4412)
  line L68 (-53.2606, 16.4412) -> (-53.2606, 16.5006)
  spline S69 degree 2 poles (-53.2606, 16.5006) (-53.1914, 16.5945) (-53.0134, 16.9455) (-52.9343, 17.158) knots 0 0 0 1 2 2 2
  spline S70 degree 2 poles (-52.9343, 17.158) (-52.8503, 17.4002) (-52.7564, 17.8006) (-52.7564, 18.0527) knots 0 0 0 1 2 2 2
  spline S71 degree 2 poles (-52.7564, 18.0527) (-52.7564, 18.2999) (-52.9343, 18.7646) (-53.1271, 18.9327) knots 0 0 0 1 2 2 2
  spline S72 degree 2 poles (-53.1271, 18.9327) (-53.31, 19.0859) (-53.7944, 19.2441) (-54.1207, 19.2441) knots 0 0 0 1 2 2 2
  spline S73 degree 2 poles (-54.1207, 19.2441) (-54.447, 19.2441) (-54.8622, 19.0661) (-55.0006, 18.898) knots 0 0 0 1 2 2 2
  spline S74 degree 2 poles (-55.0006, 18.898) (-55.1538, 18.725) (-55.2824, 18.2109) (-55.2824, 17.8995) knots 0 0 0 1 2 2 2
  spline S75 degree 2 poles (-55.2824, 17.8995) (-55.2824, 17.5634) (-55.1786, 16.896) (-55.1341, 16.6933) knots 0 0 0 1 2 2 2
  line L69 (-55.1341, 16.6933) -> (-58.278, 16.6933)
  line L70 (-58.278, 16.6933) -> (-58.278, 20.0399)
  line L71 (-58.278, 20.0399) -> (-57.5612, 20.0399)
  line L72 (-57.5612, 20.0399) -> (-57.5612, 17.4793)
  line L73 (-57.5612, 17.4793) -> (-55.9349, 17.4793)
  spline S76 degree 2 poles (-55.9349, 17.4793) (-55.9547, 17.6276) (-55.9695, 17.9143) (-55.9695, 18.033) knots 0 0 0 1 2 2 2
  spline S77 degree 2 poles (-55.9695, 18.033) (-55.9695, 18.5026) (-55.8162, 19.1502) (-55.5889, 19.4468) knots 0 0 0 1 2 2 2
  spline S78 degree 2 poles (-55.5889, 19.4468) (-55.3615, 19.7483) (-54.6694, 20.0745) (-54.1158, 20.0745) knots 0 0 0 1 2 2 2
  line L74 (-54.4766, 23.1888) -> (-54.4766, 20.8803)
  line L75 (-54.4766, 20.8803) -> (-55.2181, 20.8803)
  line L76 (-55.2181, 20.8803) -> (-55.2181, 23.1888)
  line L77 (-55.2181, 23.1888) -> (-54.4766, 23.1888)
  line L78 (-52.178, 27.4549) -> (-52.178, 24.479)
  line L79 (-52.178, 24.479) -> (-52.8008, 24.479)
  line L80 (-52.8008, 24.479) -> (-52.8008, 25.5863)
  line L81 (-52.8008, 25.5863) -> (-56.8889, 25.5863)
  line L82 (-56.8889, 25.5863) -> (-56.8889, 24.479)
  line L83 (-56.8889, 24.479) -> (-57.4475, 24.479)
  spline S79 degree 2 poles (-57.4475, 24.479) (-57.4475, 25.1068) (-57.8034, 25.7) (-58.2978, 25.7395) knots 0 0 0 1 2 2 2
  line L84 (-58.2978, 25.7395) -> (-58.2978, 26.3723)
  line L85 (-58.2978, 26.3723) -> (-52.8008, 26.3723)
  line L86 (-52.8008, 26.3723) -> (-52.8008, 27.4549)
  line L87 (-52.8008, 27.4549) -> (-52.178, 27.4549)
  line L88 (-52.178, 32.3388) -> (-52.178, 28.577)
  line L89 (-52.178, 28.577) -> (-53.0431, 28.577)
  spline S80 degree 2 poles (-53.0431, 28.577) (-53.4237, 28.9823) (-54.1306, 29.704) (-54.5112, 30.0501) knots 0 0 0 1 2 2 2
  spline S81 degree 2 poles (-54.5112, 30.0501) (-55.2774, 30.7471) (-56.1969, 31.2562) (-56.6863, 31.2562) knots 0 0 0 1 2 2 2
  spline S82 degree 2 poles (-56.6863, 31.2562) (-56.9433, 31.2562) (-57.3289, 31.098) (-57.4525, 30.9547) knots 0 0 0 1 2 2 2
  spline S83 degree 2 poles (-57.4525, 30.9547) (-57.5761, 30.8113) (-57.6996, 30.4357) (-57.6996, 30.2083) knots 0 0 0 1 2 2 2
  spline S84 degree 2 poles (-57.6996, 30.2083) (-57.6996, 29.9908) (-57.5909, 29.5459) (-57.5068, 29.3432) knots 0 0 0 1 2 2 2
  spline S85 degree 2 poles (-57.5068, 29.3432) (-57.4376, 29.1702) (-57.2399, 28.8489) (-57.1707, 28.75) knots 0 0 0 1 2 2 2
  line L90 (-57.1707, 28.75) -> (-57.1707, 28.7055)
  line L91 (-57.1707, 28.7055) -> (-58.0407, 28.7055)
  spline S86 degree 2 poles (-58.0407, 28.7055) (-58.1643, 28.9576) (-58.4065, 29.8622) (-58.4065, 30.2676) knots 0 0 0 1 2 2 2
  spline S87 degree 2 poles (-58.4065, 30.2676) (-58.4065, 31.1228) (-57.5019, 32.0867) (-56.7308, 32.0867) knots 0 0 0 1 2 2 2
  spline S88 degree 2 poles (-56.7308, 32.0867) (-56.3699, 32.0867) (-55.7668, 31.9186) (-55.5098, 31.7703) knots 0 0 0 1 2 2 2
  spline S89 degree 2 poles (-55.5098, 31.7703) (-55.2428, 31.622) (-54.7188, 31.192) (-54.4667, 30.9547) knots 0 0 0 1 2 2 2
  spline S90 degree 2 poles (-54.4667, 30.9547) (-54.0466, 30.5691) (-53.1469, 29.625) (-52.8849, 29.3432) knots 0 0 0 1 2 2 2
  line L92 (-52.8849, 29.3432) -> (-52.8849, 32.3388)
  line L93 (-52.8849, 32.3388) -> (-52.178, 32.3388)
  line L94 (-52.178, 36.9163) -> (-52.178, 33.1545)
  line L95 (-52.178, 33.1545) -> (-53.0431, 33.1545)
  spline S91 degree 2 poles (-53.0431, 33.1545) (-53.4237, 33.5598) (-54.1306, 34.2815) (-54.5112, 34.6275) knots 0 0 0 1 2 2 2
  spline S92 degree 2 poles (-54.5112, 34.6275) (-55.2774, 35.3245) (-56.1969, 35.8337) (-56.6863, 35.8337) knots 0 0 0 1 2 2 2
  spline S93 degree 2 poles (-56.6863, 35.8337) (-56.9433, 35.8337) (-57.3289, 35.6755) (-57.4525, 35.5322) knots 0 0 0 1 2 2 2
  spline S94 degree 2 poles (-57.4525, 35.5322) (-57.5761, 35.3888) (-57.6996, 35.0131) (-57.6996, 34.7857) knots 0 0 0 1 2 2 2
  spline S95 degree 2 poles (-57.6996, 34.7857) (-57.6996, 34.5682) (-57.5909, 34.1233) (-57.5068, 33.9207) knots 0 0 0 1 2 2 2
  spline S96 degree 2 poles (-57.5068, 33.9207) (-57.4376, 33.7476) (-57.2399, 33.4263) (-57.1707, 33.3275) knots 0 0 0 1 2 2 2
  line L96 (-57.1707, 33.3275) -> (-57.1707, 33.283)
  line L97 (-57.1707, 33.283) -> (-58.0407, 33.283)
  spline S97 degree 2 poles (-58.0407, 33.283) (-58.1643, 33.5351) (-58.4065, 34.4397) (-58.4065, 34.8451) knots 0 0 0 1 2 2 2
  spline S98 degree 2 poles (-58.4065, 34.8451) (-58.4065, 35.7002) (-57.5019, 36.6642) (-56.7308, 36.6642) knots 0 0 0 1 2 2 2
  spline S99 degree 2 poles (-56.7308, 36.6642) (-56.3699, 36.6642) (-55.7668, 36.4961) (-55.5098, 36.3478) knots 0 0 0 1 2 2 2
  spline S100 degree 2 poles (-55.5098, 36.3478) (-55.2428, 36.1995) (-54.7188, 35.7694) (-54.4667, 35.5322) knots 0 0 0 1 2 2 2
  spline S101 degree 2 poles (-54.4667, 35.5322) (-54.0466, 35.1466) (-53.1469, 34.2024) (-52.8849, 33.9207) knots 0 0 0 1 2 2 2
  line L98 (-52.8849, 33.9207) -> (-52.8849, 36.9163)
  line L99 (-52.8849, 36.9163) -> (-52.178, 36.9163)
  spline S102 degree 2 poles (-44.008, -28.9825) (-43.5532, -28.9825) (-42.8562, -29.3285) (-42.6288, -29.6152) knots 0 0 0 1 2 2 2
  spline S103 degree 2 poles (-42.6288, -29.6152) (-42.3619, -29.9613) (-42.1345, -30.7473) (-42.1345, -31.3701) knots 0 0 0 1 2 2 2
  line L100 (-42.1345, -31.3701) -> (-42.1345, -33.12)
  line L101 (-42.1345, -33.12) -> (-48.2345, -33.12)
  line L102 (-48.2345, -33.12) -> (-48.2345, -31.5036)
  spline S104 degree 2 poles (-48.2345, -31.5036) (-48.2345, -30.8511) (-48.1505, -30.1985) (-47.9873, -29.902) knots 0 0 0 1 2 2 2
  spline S105 degree 2 poles (-47.9873, -29.902) (-47.8143, -29.5708) (-47.2459, -29.2692) (-46.8603, -29.2692) knots 0 0 0 1 2 2 2
  spline S106 degree 2 poles (-46.8603, -29.2692) (-46.4302, -29.2692) (-45.748, -29.724) (-45.5553, -30.1244) knots 0 0 0 1 2 2 2
  line L103 (-45.5553, -30.1244) -> (-45.5256, -30.1244)
  spline S107 degree 2 poles (-45.5256, -30.1244) (-45.3773, -29.5806) (-44.5913, -28.9825) (-44.008, -28.9825) knots 0 0 0 1 2 2 2
  spline S108 degree 2 poles (-43.9734, -29.8278) (-44.3194, -29.8278) (-44.7643, -30.0255) (-44.9225, -30.3221) knots 0 0 0 1 2 2 2
  spline S109 degree 2 poles (-44.9225, -30.3221) (-45.0214, -30.5149) (-45.0807, -30.9697) (-45.0807, -31.3899) knots 0 0 0 1 2 2 2
  line L104 (-45.0807, -31.3899) -> (-45.0807, -32.3093)
  line L105 (-45.0807, -32.3093) -> (-42.8266, -32.3093)
  line L106 (-42.8266, -32.3093) -> (-42.8266, -31.6519)
  spline S110 degree 2 poles (-42.8266, -31.6519) (-42.8266, -31.118) (-42.9254, -30.505) (-43.0836, -30.2678) knots 0 0 0 1 2 2 2
  spline S111 degree 2 poles (-43.0836, -30.2678) (-43.2467, -30.0404) (-43.6521, -29.8278) (-43.9734, -29.8278) knots 0 0 0 1 2 2 2
  spline S112 degree 2 poles (-46.7466, -30.1145) (-46.9641, -30.1145) (-47.2903, -30.2628) (-47.3843, -30.4259) knots 0 0 0 1 2 2 2
  spline S113 degree 2 poles (-47.3843, -30.4259) (-47.493, -30.6237) (-47.5424, -31.1032) (-47.5424, -31.5332) knots 0 0 0 1 2 2 2
  line L107 (-47.5424, -31.5332) -> (-47.5424, -32.3093)
  line L108 (-47.5424, -32.3093) -> (-45.7579, -32.3093)
  line L109 (-45.7579, -32.3093) -> (-45.7579, -31.3899)
  spline S114 degree 2 poles (-45.7579, -31.3899) (-45.7579, -31.0092) (-45.837, -30.6484) (-45.9606, -30.4556) knots 0 0 0 1 2 2 2
  spline S115 degree 2 poles (-45.9606, -30.4556) (-46.0792, -30.2678) (-46.4599, -30.1145) (-46.7466, -30.1145) knots 0 0 0 1 2 2 2
  line L110 (-42.1345, -24.6769) -> (-42.1345, -25.4481)
  line L111 (-42.1345, -25.4481) -> (-42.6387, -25.4481)
  spline S116 degree 2 poles (-42.6387, -25.4481) (-42.3273, -25.804) (-42.006, -26.4417) (-42.006, -26.8371) knots 0 0 0 1 2 2 2
  spline S117 degree 2 poles (-42.006, -26.8371) (-42.006, -27.1337) (-42.2037, -27.6626) (-42.4163, -27.8554) knots 0 0 0 1 2 2 2
  spline S118 degree 2 poles (-42.4163, -27.8554) (-42.6288, -28.0532) (-43.2764, -28.2707) (-43.7411, -28.2707) knots 0 0 0 1 2 2 2
  line L112 (-43.7411, -28.2707) -> (-46.712, -28.2707)
  line L113 (-46.712, -28.2707) -> (-46.712, -27.4995)
  line L114 (-46.712, -27.4995) -> (-44.1019, -27.4995)
  spline S119 degree 2 poles (-44.1019, -27.4995) (-43.7361, -27.4995) (-43.2566, -27.4451) (-43.0787, -27.3512) knots 0 0 0 1 2 2 2
  spline S120 degree 2 poles (-43.0787, -27.3512) (-42.9007, -27.2573) (-42.7376, -26.936) (-42.7376, -26.6344) knots 0 0 0 1 2 2 2
  spline S121 degree 2 poles (-42.7376, -26.6344) (-42.7376, -26.3527) (-43.0589, -25.715) (-43.2912, -25.4481) knots 0 0 0 1 2 2 2
  line L115 (-43.2912, -25.4481) -> (-46.712, -25.4481)
  line L116 (-46.712, -25.4481) -> (-46.712, -24.6769)
  line L117 (-46.712, -24.6769) -> (-42.1345, -24.6769)
  spline S122 degree 2 poles (-42.0455, -22.1756) (-42.0455, -22.8034) (-42.7623, -23.5103) (-43.5384, -23.5103) knots 0 0 0 1 2 2 2
  line L118 (-43.5384, -23.5103) -> (-46.0743, -23.5103)
  line L119 (-46.0743, -23.5103) -> (-46.0743, -24.0293)
  line L120 (-46.0743, -24.0293) -> (-46.712, -24.0293)
  line L121 (-46.712, -24.0293) -> (-46.712, -23.5103)
  line L122 (-46.712, -23.5103) -> (-48.0269, -23.5103)
  line L123 (-48.0269, -23.5103) -> (-48.0269, -22.7391)
  line L124 (-48.0269, -22.7391) -> (-46.712, -22.7391)
  line L125 (-46.712, -22.7391) -> (-46.712, -21.3204)
  line L126 (-46.712, -21.3204) -> (-46.0743, -21.3204)
  line L127 (-46.0743, -21.3204) -> (-46.0743, -22.7391)
  line L128 (-46.0743, -22.7391) -> (-43.8943, -22.7391)
  spline S123 degree 2 poles (-43.8943, -22.7391) (-43.5483, -22.7391) (-43.1676, -22.7144) (-43.0045, -22.6304) knots 0 0 0 1 2 2 2
  spline S124 degree 2 poles (-43.0045, -22.6304) (-42.8612, -22.5612) (-42.7178, -22.2498) (-42.7178, -21.9828) knots 0 0 0 1 2 2 2
  spline S125 degree 2 poles (-42.7178, -21.9828) (-42.7178, -21.795) (-42.8315, -21.444) (-42.8661, -21.3649) knots 0 0 0 1 2 2 2
  line L129 (-42.8661, -21.3649) -> (-42.8661, -21.3204)
  line L130 (-42.8661, -21.3204) -> (-42.1741, -21.3204)
  spline S126 degree 2 poles (-42.1741, -21.3204) (-42.1147, -21.5379) (-42.0455, -21.9828) (-42.0455, -22.1756) knots 0 0 0 1 2 2 2
  line L131 (-42.1345, -19.966) -> (-42.1345, -20.7371)
  line L132 (-42.1345, -20.7371) -> (-48.5064, -20.7371)
  line L133 (-48.5064, -20.7371) -> (-48.5064, -19.966)
  line L134 (-48.5064, -19.966) -> (-42.1345, -19.966)
  spline S127 degree 2 poles (-42.0307, -16.8468) (-42.0307, -17.9442) (-43.2616, -19.1503) (-44.3985, -19.1503) knots 0 0 0 1 2 2 2
  spline S128 degree 2 poles (-44.3985, -19.1503) (-45.5157, -19.1503) (-46.8405, -17.9788) (-46.8405, -17.0346) knots 0 0 0 1 2 2 2
  spline S129 degree 2 poles (-46.8405, -17.0346) (-46.8405, -16.6095) (-46.5933, -15.952) (-46.3313, -15.7098) knots 0 0 0 1 2 2 2
  spline S130 degree 2 poles (-46.3313, -15.7098) (-46.0694, -15.4626) (-45.313, -15.2007) (-44.7643, -15.2007) knots 0 0 0 1 2 2 2
  line L135 (-44.7643, -15.2007) -> (-44.3441, -15.2007)
  line L136 (-44.3441, -15.2007) -> (-44.3441, -18.3693)
  spline S131 degree 2 poles (-44.3441, -18.3693) (-43.5483, -18.3693) (-42.703, -17.5685) (-42.703, -16.8567) knots 0 0 0 1 2 2 2
  spline S132 degree 2 poles (-42.703, -16.8567) (-42.703, -16.6045) (-42.8167, -16.1152) (-42.9057, -15.9174) knots 0 0 0 1 2 2 2
  spline S133 degree 2 poles (-42.9057, -15.9174) (-43.0045, -15.7098) (-43.1775, -15.4231) (-43.2566, -15.3292) knots 0 0 0 1 2 2 2
  line L137 (-43.2566, -15.3292) -> (-43.2566, -15.2847)
  line L138 (-43.2566, -15.2847) -> (-42.4163, -15.2847)
  spline S134 degree 2 poles (-42.4163, -15.2847) (-42.3619, -15.4182) (-42.2037, -15.8235) (-42.1592, -15.9817) knots 0 0 0 1 2 2 2
  spline S135 degree 2 poles (-42.1592, -15.9817) (-42.095, -16.2041) (-42.0307, -16.5699) (-42.0307, -16.8468) knots 0 0 0 1 2 2 2
  spline S136 degree 2 poles (-44.9324, -15.952) (-45.2438, -15.9619) (-45.6986, -16.0904) (-45.8518, -16.214) knots 0 0 0 1 2 2 2
  spline S137 degree 2 poles (-45.8518, -16.214) (-46.0249, -16.3475) (-46.2078, -16.7677) (-46.2078, -17.0791) knots 0 0 0 1 2 2 2
  spline S138 degree 2 poles (-46.2078, -17.0791) (-46.2078, -17.3856) (-46.0249, -17.8156) (-45.8469, -17.9936) knots 0 0 0 1 2 2 2
  spline S139 degree 2 poles (-45.8469, -17.9936) (-45.664, -18.1666) (-45.2241, -18.3446) (-44.9324, -18.3693) knots 0 0 0 1 2 2 2
  line L139 (-44.9324, -18.3693) -> (-44.9324, -15.952)
  line L140 (-45.8865, -11.9925) -> (-45.8865, -12.032)
  spline S140 degree 2 poles (-45.8865, -12.032) (-45.9112, -12.121) (-45.9211, -12.3138) (-45.9211, -12.4473) knots 0 0 0 1 2 2 2
  spline S141 degree 2 poles (-45.9211, -12.4473) (-45.9211, -12.7587) (-45.6492, -13.3716) (-45.3822, -13.6485) knots 0 0 0 1 2 2 2
  line L141 (-45.3822, -13.6485) -> (-42.1345, -13.6485)
  line L142 (-42.1345, -13.6485) -> (-42.1345, -14.4196)
  line L143 (-42.1345, -14.4196) -> (-46.712, -14.4196)
  line L144 (-46.712, -14.4196) -> (-46.712, -13.6485)
  line L145 (-46.712, -13.6485) -> (-46.0298, -13.6485)
  spline S142 degree 2 poles (-46.0298, -13.6485) (-46.4055, -13.2283) (-46.712, -12.6005) (-46.712, -12.3039) knots 0 0 0 1 2 2 2
  spline S143 degree 2 poles (-46.712, -12.3039) (-46.712, -12.1853) (-46.7021, -12.0666) (-46.6873, -11.9925) knots 0 0 0 1 2 2 2
  line L146 (-46.6873, -11.9925) -> (-45.8865, -11.9925)
  line L147 (-42.1345, -3.4851) -> (-42.1345, -4.2958)
  line L148 (-42.1345, -4.2958) -> (-47.3892, -4.2958)
  line L149 (-47.3892, -4.2958) -> (-43.8152, -5.8875)
  line L150 (-43.8152, -5.8875) -> (-43.8152, -6.3819)
  line L151 (-43.8152, -6.3819) -> (-47.3892, -7.9588)
  line L152 (-47.3892, -7.9588) -> (-42.1345, -7.9588)
  line L153 (-42.1345, -7.9588) -> (-42.1345, -8.7151)
  line L154 (-42.1345, -8.7151) -> (-48.2345, -8.7151)
  line L155 (-48.2345, -8.7151) -> (-48.2345, -7.6078)
  line L156 (-48.2345, -7.6078) -> (-44.8385, -6.0853)
  line L157 (-44.8385, -6.0853) -> (-48.2345, -4.6122)
  line L158 (-48.2345, -4.6122) -> (-48.2345, -3.4851)
  line L159 (-48.2345, -3.4851) -> (-42.1345, -3.4851)
  spline S144 degree 2 poles (-42.6189, 0.2421) (-42.5497, 0.1482) (-42.3026, -0.1682) (-42.2284, -0.3165) knots 0 0 0 1 2 2 2
  spline S145 degree 2 poles (-42.2284, -0.3165) (-42.1197, -0.5191) (-42.006, -0.8998) (-42.006, -1.2458) knots 0 0 0 1 2 2 2
  spline S146 degree 2 poles (-42.006, -1.2458) (-42.006, -1.5276) (-42.2185, -2.0367) (-42.4113, -2.2295) knots 0 0 0 1 2 2 2
  spline S147 degree 2 poles (-42.4113, -2.2295) (-42.5992, -2.4124) (-43.1528, -2.6349) (-43.4593, -2.6349) knots 0 0 0 1 2 2 2
  spline S148 degree 2 poles (-43.4593, -2.6349) (-43.9339, -2.6349) (-44.6061, -2.2344) (-44.7989, -1.7994) knots 0 0 0 1 2 2 2
  spline S149 degree 2 poles (-44.7989, -1.7994) (-44.9769, -1.4139) (-45.1104, -0.3659) (-45.145, 0.2421) knots 0 0 0 1 2 2 2
  line L160 (-45.145, 0.2421) -> (-45.2933, 0.2421)
  spline S150 degree 2 poles (-45.2933, 0.2421) (-45.5602, 0.2421) (-45.8914, 0.079) (-45.9853, -0.0693) knots 0 0 0 1 2 2 2
  spline S151 degree 2 poles (-45.9853, -0.0693) (-46.0792, -0.2176) (-46.1386, -0.6427) (-46.1386, -0.8701) knots 0 0 0 1 2 2 2
  spline S152 degree 2 poles (-46.1386, -0.8701) (-46.1386, -1.137) (-45.9804, -1.8588) (-45.8271, -2.2196) knots 0 0 0 1 2 2 2
  line L161 (-45.8271, -2.2196) -> (-45.8271, -2.2641)
  line L162 (-45.8271, -2.2641) -> (-46.6131, -2.2641)
  spline S153 degree 2 poles (-46.6131, -2.2641) (-46.6724, -2.0515) (-46.8207, -1.2557) (-46.8207, -0.8652) knots 0 0 0 1 2 2 2
  spline S154 degree 2 poles (-46.8207, -0.8652) (-46.8207, -0.3906) (-46.6724, 0.257) (-46.4796, 0.514) knots 0 0 0 1 2 2 2
  spline S155 degree 2 poles (-46.4796, 0.514) (-46.2918, 0.7661) (-45.6937, 1.0133) (-45.2636, 1.0133) knots 0 0 0 1 2 2 2
  line L163 (-45.2636, 1.0133) -> (-42.1345, 1.0133)
  line L164 (-42.1345, 1.0133) -> (-42.1345, 0.2421)
  line L165 (-42.1345, 0.2421) -> (-42.6189, 0.2421)
  line L166 (-43.2616, 0.2421) -> (-44.532, 0.2421)
  spline S156 degree 2 poles (-44.532, 0.2421) (-44.5073, -0.0347) (-44.4232, -0.8701) (-44.3441, -1.1321) knots 0 0 0 1 2 2 2
  spline S157 degree 2 poles (-44.3441, -1.1321) (-44.2502, -1.4386) (-43.8597, -1.839) (-43.5137, -1.839) knots 0 0 0 1 2 2 2
  spline S158 degree 2 poles (-43.5137, -1.839) (-43.1182, -1.839) (-42.7178, -1.3941) (-42.7178, -0.969) knots 0 0 0 1 2 2 2
  spline S159 degree 2 poles (-42.7178, -0.969) (-42.7178, -0.6081) (-43.0292, -0.0149) (-43.2616, 0.2421) knots 0 0 0 1 2 2 2
  spline S160 degree 2 poles (-42.0455, 3.48) (-42.0455, 2.8522) (-42.7623, 2.1453) (-43.5384, 2.1453) knots 0 0 0 1 2 2 2
  line L167 (-43.5384, 2.1453) -> (-46.0743, 2.1453)
  line L168 (-46.0743, 2.1453) -> (-46.0743, 1.6262)
  line L169 (-46.0743, 1.6262) -> (-46.712, 1.6262)
  line L170 (-46.712, 1.6262) -> (-46.712, 2.1453)
  line L171 (-46.712, 2.1453) -> (-48.0269, 2.1453)
  line L172 (-48.0269, 2.1453) -> (-48.0269, 2.9164)
  line L173 (-48.0269, 2.9164) -> (-46.712, 2.9164)
  line L174 (-46.712, 2.9164) -> (-46.712, 4.3352)
  line L175 (-46.712, 4.3352) -> (-46.0743, 4.3352)
  line L176 (-46.0743, 4.3352) -> (-46.0743, 2.9164)
  line L177 (-46.0743, 2.9164) -> (-43.8943, 2.9164)
  spline S161 degree 2 poles (-43.8943, 2.9164) (-43.5483, 2.9164) (-43.1676, 2.9412) (-43.0045, 3.0252) knots 0 0 0 1 2 2 2
  spline S162 degree 2 poles (-43.0045, 3.0252) (-42.8612, 3.0944) (-42.7178, 3.4058) (-42.7178, 3.6728) knots 0 0 0 1 2 2 2
  spline S163 degree 2 poles (-42.7178, 3.6728) (-42.7178, 3.8606) (-42.8315, 4.2116) (-42.8661, 4.2907) knots 0 0 0 1 2 2 2
  line L178 (-42.8661, 4.2907) -> (-42.8661, 4.3352)
  line L179 (-42.8661, 4.3352) -> (-42.1741, 4.3352)
  spline S164 degree 2 poles (-42.1741, 4.3352) (-42.1147, 4.1177) (-42.0455, 3.6728) (-42.0455, 3.48) knots 0 0 0 1 2 2 2
  line L180 (-45.8865, 7.3308) -> (-45.8865, 7.2912)
  spline S165 degree 2 poles (-45.8865, 7.2912) (-45.9112, 7.2023) (-45.9211, 7.0095) (-45.9211, 6.876) knots 0 0 0 1 2 2 2
  spline S166 degree 2 poles (-45.9211, 6.876) (-45.9211, 6.5646) (-45.6492, 5.9516) (-45.3822, 5.6748) knots 0 0 0 1 2 2 2
  line L181 (-45.3822, 5.6748) -> (-42.1345, 5.6748)
  line L182 (-42.1345, 5.6748) -> (-42.1345, 4.9036)
  line L183 (-42.1345, 4.9036) -> (-46.712, 4.9036)
  line L184 (-46.712, 4.9036) -> (-46.712, 5.6748)
  line L185 (-46.712, 5.6748) -> (-46.0298, 5.6748)
  spline S167 degree 2 poles (-46.0298, 5.6748) (-46.4055, 6.095) (-46.712, 6.7228) (-46.712, 7.0194) knots 0 0 0 1 2 2 2